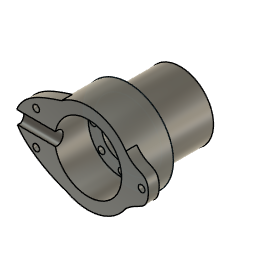
BaseVeleta v1 (Autodesk Fusion 360 design; units mm, degrees)
Autodesk Fusion 360 part; units mm, degrees
sketch "Boceto5" plane through (0, 0, 0) normal (0, 1, 0) x (1, 0, 0)
  circle A0 centre (0, 0) radius 12
  circle A1 centre (0, 0) radius 20
  line L0 (0, -18) -> (0, 20) construction
  line L1 (0, 20) -> (22, 0) construction
  line L2 (22, 0) -> (-21, 0) construction
  circle A2 centre (0, -17) radius 2
  circle A3 centre (12.0208, -12.0208) radius 2
  circle A4 centre (17, 0) radius 2
  circle A5 centre (12.0208, 12.0208) radius 2
  circle A6 centre (0, 17) radius 2
  circle A7 centre (-12.0208, 12.0208) radius 2
  circle A8 centre (-17, 0) radius 2
  circle A9 centre (-12.0208, -12.0208) radius 2
  dimension "d1" = 24
  dimension "d2" = 40
  dimension "d3" = 8
  dimension "d4" = 4
  dimension "d5" = 17
  dimension "d7" = 360
  constraint coincident A0.centre A1.centre
  constraint concentric A0 A1
  constraint vertical L0
  constraint horizontal L2
  constraint coincident L0 A2.centre
  measures "d1" diameter of A0
  measures "d2" diameter of A1
  measures "d3" distance of A0 A1
  measures "d4" diameter of A2
  measures "d5" distance of A0.centre A2.centre
extrude "Extruir1" add sketch "Boceto5" along normal blind 35
ref_plane "PlanoDeObra1" through (0, 27.7, 0) normal (0, 1, 0) x (1, 0, 0)
sketch "Boceto6" plane through (0, 27.7, 0) normal (0, 1, 0) x (1, 0, 0)
  circle A0 centre (0, 0) radius 13.2354
  circle A1 centre (0, 0) radius 5
  dimension "d11" = 10
  constraint coincident A0.centre A1.centre
  constraint concentric A0 A1
  measures "d11" diameter of A1
extrude "Extruir2" add sketch "Boceto6" against normal blind 3
sketch "Boceto7" plane through (0, 0, 0) normal (0, -1, 0) x (1, 0, 0)
  circle A0 centre (-12.0208, 12.0208) radius 2
  circle A1 centre (12.0208, 12.0208) radius 2
  circle A2 centre (-12.0208, -12.0208) radius 2
  circle A3 centre (0, 0) radius 12
  circle A4 centre (17, 0) radius 2
  circle A5 centre (12.0208, -12.0208) radius 2
  circle A6 centre (-17, 0) radius 2
  circle A7 centre (0, -17) radius 2
  circle A8 centre (0, 17) radius 2
  circle A9 centre (0, 0) radius 20
  circle A10 centre (0, 0) radius 27
  circle A11 centre (0, 0) radius 12
  constraint concentric A3 A10
  constraint concentric A10 A11
extrude "Extruir3" add sketch "Boceto7" along normal blind 20 and the other way blind 4 contours A10
sketch "Boceto8" plane through (0, -20, 0) normal (0, -1, 0) x (1, 0, 0)
  circle A0 centre (0, 0) radius 20
  circle A1 centre (0, 0) radius 27
  spline S0 degree 5 poles (0.8049, -26.988) (-1.1916, -26.6528) (-5.0661, -25.9145) (-10.5223, -24.6033) (-17.129, -22.45) (-24.4438, -19.1245) (-30.9638, -15.2359) (-36.6141, -10.944) (-41.1579, -6.4179) (-43.6205, -2.0992) (-43.7018, 2.1218) (-41.8139, 6.6729) (-38.2196, 11.3661) (-32.8205, 15.2954) (-25.9465, 18.4821) (-17.9948, 21.1667) (-11.1308, 23.2874) (-5.8571, 25.0495) (-2.3066, 26.329) (-0.5226, 26.9949) knots 0 0 0 0 0 0 0.066667 0.133333 0.2 0.266667 0.333333 0.4 0.466667 0.533333 0.6 0.666667 0.733333 0.8 0.866667 0.933333 1 1 1 1 1 1
  spline S1 degree 5 poles (22.4701, -14.9698) (23.4209, -14.1205) (25.2562, -12.6285) (27.8097, -11.0079) (30.796, -9.7676) (33.7124, -8.1227) (35.6265, -5.0956) (36.3527, 0.0255) (35.6595, 4.9302) (33.5709, 7.4325) (30.4274, 8.6009) (27.3931, 9.8371) (24.9893, 11.8342) (23.3518, 13.7692) (22.5244, 14.888) knots 0 0 0 0 0 0 0.1 0.2 0.3 0.4 0.5 0.6 0.7 0.8 0.9 1 1 1 1 1 1
  line L0 (36, -3.7373) -> (36, 3.7373)
  line L1 (18.3284, -18.669) -> (26.6118, -11.2706)
  line L2 (26.1391, 10.0004) -> (18.9097, 19.7756)
  circle A2 centre (32, 0.1921) radius 2
  circle A3 centre (-31.1235, -10.1718) radius 2
  line L3 (-65, 0) -> (0, 0) construction
  line L4 (0, 0) -> (0, -32.1871) construction
  circle A4 centre (-31.1235, 10.1718) radius 2
  line L5 (-46.074, -0.0716) -> (-35.3734, 15.5371)
  circle A5 centre (0, 0) radius 27 construction
  line L6 (15.8053, -29.5065) -> (-14.1954, -24.4695)
  line L7 (-14.284, 21.8582) -> (13.2387, 32.1317)
  line L8 (-33.4619, -14.8868) -> (-46.5381, 0.3871)
  point P0 (-40, -7.2498)
  point P1 (-40.7237, 7.7327)
  point P2 (36, 0)
  dimension "d18" = 4
  dimension "d19" = 4
  dimension "d20" = 36
  dimension "d21" = 32
  dimension "d22" = 15
  dimension "d23" = 40
  dimension "d24" = 30
  dimension "d25" = 105
  constraint coincident A1 S0.start
  constraint coincident A1 S0.end
  constraint coincident A1 S1.start
  constraint coincident A1 S1.end
  constraint midpoint P2 L0
  constraint midpoint S1.start L1
  constraint midpoint S1.end L2
  constraint coincident A0.centre A1.centre
  constraint horizontal L3
  constraint perpendicular L3 L4
  constraint symmetric A3 L3 A4
  constraint midpoint P1 L5
  constraint midpoint S0.start L6
  constraint midpoint S0.end L7
  constraint midpoint P0 L8
  measures "d18" diameter of A3
  measures "d19" diameter of A2
  measures "d20" distance of P2 A0.centre
  measures "d21" horizontal distance of A2.centre A0.centre
  measures "d22" distance of P0 P1
  measures "d23" horizontal distance of P0 A0.centre
  measures "d24" angle of L6 L7
  measures "d25" angle of L5 L8
extrude "Extruir4" add sketch "Boceto8" against normal blind 6.5 contours A1 S1 | A1 S0 picked at (-33.9376, 4.4367)
ref_plane "PlanoDeObra2" through (-5, 0, 0) normal (1, 0, 0) x (0, 1, 0)
sketch "Boceto9" plane through (0, 0, 0) normal (0, -1, 0) x (1, 0, 0)
sketch "Boceto10" plane through (-5, 0, 0) normal (1, 0, 0) x (0, 1, 0)
  circle A0 centre (-19, 0) radius 4
  line L0 (-20, -23.6837) -> (-20, 21.762)
  dimension "d31" = 8
  dimension "d32" = 1
  measures "d31" diameter of A0
  measures "d32" distance of A0.centre L0
extrude "Extruir5" cut sketch "Boceto10" against normal blind 48
sketch "Boceto11" plane through (0, 4, 0) normal (0, 1, 0) x (-1, 0, 0)
  circle A0 centre (0, 0) radius 20
  circle A1 centre (0, 0) radius 27
